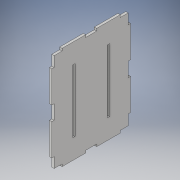
# Autodesk Inventor part: case_side
Saved by Autodesk Inventor 2019 (Build 230136000, 136)
## iProperties
Created: 2019-07-12
Part Number: case_side
Material: Generic
Document SubType Name: Modeling
Designer: Lino P
Density: 1 g/cm^3
Appearance: Default
Author: Lino P
Autodesk Inventor part; units mm, degrees
ref_plane "YZ Plane" through (0, 0, 0) normal (1, 0, 0) x (0, 1, 0)
ref_plane "XZ Plane" through (0, 0, 0) normal (0, 1, 0) x (-1, 0, 0)
ref_plane "Work Plane1" through (249, 4.2, 0) normal (1, 0, 0) x (0, 0, -1)
sketch "Sketch2" plane through (249, 4.2, 0) normal (1, 0, 0) x (0, 0, -1)
  line L0 (0, -18.2) -> (0, -58.2) projected
  line L1 (0, -18.2) -> (-3, -18.2) projected
  line L2 (-3, -58.2) -> (-3, -18.2) construction
  line L3 (0, -58.2) -> (-3, -58.2) projected
  line L4 (-3, 56) -> (-3, 53) construction
  line L5 (0, -74.2) -> (-3, -74.2) projected
  line L6 (0, 56) -> (94, 56) construction
  line L7 (94, 53) -> (94, -71.2)
  line L8 (94, -74.2) -> (0, -74.2) construction
  line L9 (0, -71.2) -> (0, 53)
  line L10 (-3, -18.2) -> (0, -18.2)
  line L11 (0, -18.2) -> (0, -58.2)
  line L12 (0, -58.2) -> (-3, -58.2)
  line L13 (-3, -58.2) -> (-3, -18.2)
  line L14 (47, 56) -> (47, -74.2) construction
  line L15 (0, -9.1) -> (94, -9.1) construction
  line L16 (94, 40) -> (94, 0)
  line L17 (97, 0) -> (97, 40) construction
  line L18 (94, 0) -> (97, 0)
  line L19 (94, -18.2) -> (94, -58.2)
  line L20 (94, -18.2) -> (97, -18.2)
  line L21 (97, -58.2) -> (97, -18.2) construction
  line L22 (94, -58.2) -> (97, -58.2)
  line L23 (97, -18.2) -> (94, -18.2)
  line L24 (94, -18.2) -> (94, -58.2)
  line L25 (94, -58.2) -> (97, -58.2)
  line L26 (97, -58.2) -> (97, -18.2)
  line L27 (94, 21.75) -> (94, 0.05)
  line L28 (97, 40) -> (94, 40)
  line L29 (94, 40) -> (94, 0.05)
  line L30 (94, 0.05) -> (97, 0.05)
  line L31 (97, 0.05) -> (97, 40)
  line L32 (0, 40) -> (0, 56) construction
  line L33 (94, 56) -> (0, 56) construction
  line L34 (0, 56) -> (0, 53) construction
  line L35 (0, 53) -> (94, 53)
  line L36 (94, 53) -> (94, 56) construction
  line L37 (10, 53) -> (40, 53)
  line L38 (40, 53) -> (40, 56)
  line L39 (40, 56) -> (10, 56)
  line L40 (10, 56) -> (10, 53)
  line L41 (84, 53) -> (54, 53)
  line L42 (54, 53) -> (54, 56)
  line L43 (54, 56) -> (84, 56)
  line L44 (84, 56) -> (84, 53)
  line L45 (10, -71.2) -> (40, -71.2)
  line L46 (40, -71.2) -> (40, -74.2)
  line L47 (40, -74.2) -> (10, -74.2)
  line L48 (10, -74.2) -> (10, -71.2)
  line L49 (84, -74.2) -> (84, -71.2)
  line L50 (84, -71.2) -> (54, -71.2)
  line L51 (54, -71.2) -> (54, -74.2)
  line L52 (54, -74.2) -> (84, -74.2)
  line L53 (0, -71.2) -> (94, -71.2)
  line L54 (0, 40) -> (0, 0) construction
  line L55 (0, 40) -> (-3, 40) construction
  line L56 (-3, 0) -> (-3, 40) construction
  line L57 (0, 0) -> (-3, 0) construction
  line L58 (-3, 0) -> (0, 0) construction
  line L59 (0, 0) -> (0, 40) construction
  line L60 (0, 40) -> (-3, 40) construction
  line L61 (-3, 40) -> (-3, 0) construction
  line L62 (0, 40) -> (-3, 40) projected
  line L63 (-3, 40) -> (0, 40)
  line L64 (0, 40) -> (0, 0)
  line L65 (0, 0) -> (-3, 0)
  line L66 (-3, 0) -> (-3, 40)
  point P0 (0, -4.2)
  point P1 (0, 21.75)
  point P2 (0, 0.05)
  point P3 (94, -4.2)
  dimension "d47" = 94
  dimension "d48" = 3
  dimension "d49" = 30
  dimension "d54" = 10
  constraints: 110 end point, 26 symmetric about line, 12 parallel, 7 perpendicular, 6 horizontal, 4 midpoint, 3 point on line, 1 coincident
  measures "d47" distance of L5.start L8.start
  measures "d48" distance of L9.end L33.end
  measures "d49" distance of L39.end L38.end
  measures "d54" distance from line of L9.end L40
extrude "Extrusion3" add sketch "Sketch2" along normal blind 3
sketch "Sketch3" plane through (252, 4.2, 0) normal (1, 0, 0) x (0, 0, -1)
  line L0 (0, -18.2) -> (-3, -18.2) construction
  line L1 (-3, -18.2) -> (-3, -58.2) construction
  line L2 (-3, -58.2) -> (0, -58.2) construction
  line L3 (0, -58.2) -> (0, -71.2) construction
  line L4 (0, -71.2) -> (10, -71.2) construction
  line L5 (10, -71.2) -> (10, -74.2) construction
  line L6 (10, -74.2) -> (40, -74.2) construction
  line L7 (40, -74.2) -> (40, -71.2) construction
  line L8 (40, -71.2) -> (54, -71.2) construction
  line L9 (54, -71.2) -> (54, -74.2) construction
  line L10 (54, -74.2) -> (84, -74.2) construction
  line L11 (84, -74.2) -> (84, -71.2) construction
  line L12 (84, -71.2) -> (94, -71.2) construction
  line L13 (94, -71.2) -> (94, -58.2) construction
  line L14 (94, -58.2) -> (97, -58.2) construction
  line L15 (97, -58.2) -> (97, -18.2) construction
  line L16 (97, -18.2) -> (94, -18.2) construction
  line L17 (94, -18.2) -> (94, 0.05) construction
  line L18 (94, 0.05) -> (97, 0.05) construction
  line L19 (97, 0.05) -> (97, 40) construction
  line L20 (97, 40) -> (94, 40) construction
  line L21 (94, 40) -> (94, 53) construction
  line L22 (94, 53) -> (84, 53) construction
  line L23 (84, 53) -> (84, 56) construction
  line L24 (84, 56) -> (54, 56) construction
  line L25 (54, 56) -> (54, 53) construction
  line L26 (54, 53) -> (40, 53) construction
  line L27 (40, 53) -> (40, 56) construction
  line L28 (40, 56) -> (10, 56) construction
  line L29 (10, 56) -> (10, 53) construction
  line L30 (10, 53) -> (0, 53) construction
  line L31 (0, 53) -> (0, 40) construction
  line L32 (0, 40) -> (-3, 40) construction
  line L33 (-3, 40) -> (-3, 0) construction
  line L34 (-3, 0) -> (0, 0) construction
  line L35 (0, 0) -> (0, -18.2) construction
  line L36 (47, 53) -> (47, -71.2) construction
  line L37 (0, -9.1) -> (94, -9.075) construction
  line L38 (23.5, -49.0934) -> (26.5, -49.0934)
  line L39 (26.5, -49.0934) -> (26.5, 30.9066)
  line L40 (26.5, 30.9066) -> (23.5, 30.9066)
  line L41 (23.5, 30.9066) -> (23.5, -49.0934)
  line L42 (23.5, -49.0934) -> (26.5, 30.9066) construction
  line L43 (26.5, -49.0934) -> (23.5, 30.9066) construction
  line L44 (70.5, -49.0934) -> (67.5, -49.0934)
  line L45 (67.5, -49.0934) -> (67.5, 30.9066)
  line L46 (67.5, 30.9066) -> (70.5, 30.9066)
  line L47 (70.5, 30.9066) -> (70.5, -49.0934)
  line L48 (70.5, -49.0934) -> (67.5, 30.9066) construction
  line L49 (67.5, -49.0934) -> (70.5, 30.9066) construction
  point P0 (0, -4.2)
  point P1 (25, -9.0934)
  point P2 (69, -9.0934)
  dimension "d55" = 3
  dimension "d56" = 80
  constraints: 28 end point, 8 midpoint, 5 symmetric about line, 2 parallel, 1 horizontal, 1 perpendicular, 1 point on line
  measures "d55" distance of L40.end L39.end
  measures "d56" distance of L38.start L40.end
extrude "Extrusion4" cut sketch "Sketch3" along normal mid plane 10
body "Solid1"
